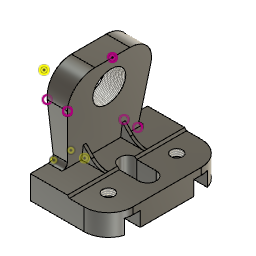
Surprise Checkpoint Q6 v1 (Autodesk Fusion 360 design; units mm, degrees)
Autodesk Fusion 360 part; units mm, degrees
note: some values were not read from the file. Chosen so that the rebuilt part matches the saved one: which face or edge a step refers to; the sign of a taper; which pieces of a blend or face edit are solid.
sketch "Sketch1" plane through (0, 0, 0) normal (0, 1, 0) x (1, 0, 0)
  line L0 (0, 0) -> (0, -24)
  line L1 (0, 0) -> (80, 0)
  line L2 (80, 0) -> (80, -22)
  line L3 (80, -22) -> (40, -22)
  line L4 (0, -24) -> (38, -24)
  line L5 (38, -24) -> (40, -22)
  dimension "d1" = 24
  dimension "d2" = 80
  dimension "d3" = 22
  dimension "d4" = 40
  dimension "d5" = 38
  constraint coincident L0.start L1.start
  constraint vertical L0
  constraint perpendicular L0 L1
  constraint perpendicular L1 L2
  constraint perpendicular L2 L3
  constraint perpendicular L0 L4
  measures "d1" distance of L0.start L0.end
  measures "d2" distance of L0.start L1.end
  measures "d3" distance of L1.end L2.end L0.start
  measures "d4" distance of L2.end L3.end L0.start
  measures "d5" distance of L0.end L4.end
extrude "Extrude1" add sketch "Sketch1" along normal blind 120 makes body 1
fillet "Fillet1" radius 25 2 edges at (80, 0, 11) (80, 120, 11) on bodies 1
hole "Hole1" at (55, 25, 22) direction (0, 0, -1) diameter 12.023 depth 7 tip angle 180 bodies 1
thread "Thread1" "ISO Metric profile 14.0 M14x2 6H"
hole "Hole2" at (55, 95, 22) direction (0, 0, -1) diameter 12.023 depth 7 tip angle 180 bodies 1
thread "Thread2" "ISO Metric profile 14.0 M14x2 6H"
ref_plane "WorkPlane1" through (27.5, 60, 12) normal (0, -1, 0) x (-1, 0, 0)
sketch "Sketch2" plane through (27.5, 60, 12) normal (0, -1, 0) x (1, 0, 0)
  line L0 (27.5, 10) -> (27.5, -12)
  line L1 (27.5, -12) -> (-27.5, -12)
  line L2 (-27.5, -12) -> (-27.5, 12)
  line L3 (-27.5, 12) -> (10.5, 12)
  line L4 (10.5, 12) -> (12.5, 10)
  line L5 (12.5, 10) -> (27.5, 10)
  line L6 (-27.5, -12) -> (-27.5, 97)
  line L7 (-27.5, 97) -> (-3.5, 97)
  line L8 (-27.5, 12) -> (35, 12) construction
  line L9 (-3.5, 97) -> (76.6186, 97) construction
  line L10 (-3.5, 97) -> (82.0862, 97) construction
  line L11 (-3.5, 97) -> (-13.4998, 12)
  line L12 (-3.5, 97) -> (-89.0862, 97) construction
  dimension "d21" = 109
  dimension "d25" = 83.29
  constraint coincident L1.end L2.start
  constraint perpendicular L3 L6
  constraint perpendicular L6 L7
  constraint coincident L2.end L3.start
  constraint perpendicular L2 L8
  constraint horizontal L9
  constraint horizontal L10
  constraint horizontal L12
  constraint coincident L3 L11.end
  measures "d21" distance of L1.end L6.end
  measures "d25" angle of L11 L12
ref_plane "WorkPlane2" through (0, 60, 12) normal (-1, 0, 0) x (0, 0, 1)
sketch "Sketch3" plane through (0, 60, 12) normal (-1, 0, 0) x (0, 1, 0)
ref_plane "WorkPlane3" through (19, 60, 24) normal (0, 0, 1) x (1, 0, 0)
sketch "Sketch4" plane through (0, 0, 24) normal (0, 0, 1) x (-1, 0, 0)
  line L0 (0, 0) -> (-38, 0)
  line L1 (-38, 0) -> (-38, -120)
  line L2 (-38, -120) -> (0, -120)
  line L3 (0, -120) -> (0, 0)
  line L4 (-14.0002, -60) -> (-14.0002, 0)
  line L5 (0, 0) -> (0, -60)
  line L6 (0, -60) -> (0, -30)
  line L7 (0, -60) -> (0, -30)
  point P0 (-14.0002, -60)
  point P1 (0, -60)
  point P2 (0, 0)
  constraint coincident P0 L4.start
  constraint coincident L0 L4.end
  constraint perpendicular L0 L4
  constraint coincident P2 L0.start
  constraint coincident P1 L5.end
  constraint midpoint L5 L6.end
  constraint parallel L6 L7
sketch "Sketch5" plane through (0, 60, 12) normal (-1, 0, 0) x (0, 1, 0)
ref_plane "WorkPlane4" through (24, 60, 109) normal (0, 0, 1) x (1, 0, 0)
sketch "Sketch6" plane through (24, 60, 109) normal (0, 0, 1) x (1, 0, 0)
  point P0 (-24, -45.9998)
ref_plane "WorkPlane5" through (0, 14.0002, 109) normal (0, 0.993151, 0.116837) x (-1, 0, 0)
sketch "Sketch7" plane through (0, 14.0002, 109) normal (0, 0.993151, 0.116837) x (-1, 0, 0)
  point P0 (0, -85.5862)
sweep "Sweep1" add profiles "Sketch2" path "Sketch4" along L5 for 0.59993 of its length starting at (0, 0, 24) heading (0, 1, 0) section 1 contours L3 L6 L7 L11 bodies 1
draft "Draft1" angle 6.71 neutral plane through (0, 14.0002, 109) pull (0, -0.993151, -0.116837) 1 faces at (12.6667, 24.0042, 80.6667) on bodies 1
fillet "Fillet2" radius 25 1 edges at (12, 14, 109) on bodies 1
ref_plane "WorkPlane6" through (24, 60, 109) normal (0, -1, 0) x (1, 0, 0)
sketch "Sketch8" plane through (11.0241, 0, -1.2969) normal (0.993151, 0, -0.116839) x (0, 1, 0)
  ellipse E0 centre (42.1135, 85.8852) end of major axis (42.1135, 111.0576) minor radius 25 (42.1135, 111.0576) -> (17.2848, 82.944) ccw
  line L0 (60, 111.0576) -> (42.1135, 111.0576)
mirror "Mirror1" about plane through (24, 60, 109) normal (0, -1, 0) of bodies 1 makes body 2
combine "Combine1" operation add target body 1 tool bodies 2
sketch "Sketch9" plane through (0, 0, 24) normal (0, 0, 1) x (-1, 0, 0)
  line L0 (0, -96.0002) -> (-14.0002, -96.0002)
sketch "Sketch10" plane through (11.0241, 0, -1.2969) normal (0.993151, 0, -0.116839) x (0, 1, 0)
  ellipse E0 centre (42.1135, 85.8852) end of major axis (42.1135, 111.0576) minor radius 25 (42.1135, 111.0576) -> (17.2848, 82.944) ccw
  line L0 (96.0002, 25.4714) -> (102.7152, 82.944)
  ellipse E1 centre (77.8865, 85.8852) end of major axis (77.8865, 111.0576) minor radius 25 (102.7152, 82.944) -> (77.8865, 111.0576) ccw
  line L1 (77.8865, 111.0576) -> (42.1135, 111.0576)
  point P0 (41.5, 25.4714)
sketch "Sketch11" plane through (0, 0, 24) normal (0, 0, 1) x (-1, 0, 0)
sketch "Sketch12" plane through (0, 0, 22) normal (0, 0, 1) x (-1, 0, 0)
  circle A0 centre (-55, -95) radius 6.0113
  circle A1 centre (-55, -25) radius 6.0113
  arc A2 (-80, -95) -> (-55, -120) centre (-55, -95) ccw
  line L0 (-55, -120) -> (-40, -120)
  line L1 (-40, 0) -> (-55, 0)
  arc A3 (-55, 0) -> (-80, -25) centre (-55, -25) ccw
  line L2 (-80, -25) -> (-80, -95)
  arc A4 (-60, -51) -> (-60, -69) centre (-60, -60) ccw
  line L3 (-60, -51) -> (-57.6575, -51)
  line L4 (-57.6575, -51) -> (-40, -51)
  line L5 (-60, -69) -> (-40, -69)
  arc A5 (-40, -69) -> (-40, -51) centre (-40, -60) ccw
  dimension "d48" = 9
  constraint tangent A4 L5
  measures "d48" radius of A4
extrude "Extrude2" cut sketch "Sketch12" along normal blind 2 and the other way blind 22 contours A4 L3 L4 L5 A5 bodies 1
sketch "Sketch13" plane through (0, 0, 0) normal (-1, 0, 0) x (0, -1, 0)
  arc A0 (-17.2848, 81.079) -> (-42.1135, 109) centre (-42.1135, 84) ccw
  line L0 (-42.1135, 109) -> (-77.8865, 109)
  arc A1 (-77.8865, 109) -> (-102.7152, 81.079) centre (-77.8865, 84) ccw
  line L1 (-102.7152, 81.079) -> (-96.0002, 24)
hole "Hole3" at (0, 60.0039, 81.6923) direction (1, 0, 0) diameter 33.526 depth 30 tip angle 180 bodies 1
thread "Thread3" "ISO Metric profile 35.0 M35x1.5 6H"
fillet "Fillet3" radius 5 1 edges at (7.0001, 96.0002, 24) on bodies 1
fillet "Fillet3" radius 5 1 edges at (7.0001, 23.9998, 24) on bodies 1
sketch "Sketch14" plane through (0, 26.4571, 3.1126) normal (0, -0.993151, -0.116839) x (1, 0, 0)
ref_plane "WorkPlane7" through (14.0002, 41.5, 24) normal (0.993151, 0, -0.116839) x (0, 1, 0)
sketch "Sketch15" plane through (14.0002, 41.5, 24) normal (0.993151, 0, -0.116839) x (0, 1, 0)
ref_plane "WorkPlane8" through (0, 24, 24) normal (-1, 0, 0) x (0, -1, 0)
sketch "Sketch16" plane through (0, 24, 24) normal (-1, 0, 0) x (0, 1, 0)
  point P0 (17.5, 0)
sketch "Sketch17" plane through (14.0002, 41.5, 24) normal (0.993151, 0, -0.116839) x (0, 1, 0)
ref_plane "WorkPlane9" through (0, 41.5, 24) normal (0, 1, 0) x (-1, 0, 0)
sketch "Sketch18" plane through (0, 41.5, 24) normal (0, 1, 0) x (1, 0, 0)
  point P0 (14.0002, 0)
sketch "Sketch19" plane through (0, 0, 24) normal (0, 0, 1) x (1, 0, 0)
sketch "Sketch20" plane through (0, 0, 24) normal (0, 0, 1) x (1, 0, 0)
sketch "Sketch21" plane through (0, 41.5, 24) normal (0, 1, 0) x (1, 0, 0)
  line L0 (14.0002, 0) -> (38, 0)
  line L1 (26.4, 0) -> (26.4, 24)
  line L2 (38, 0) -> (38, 23.5536)
  line L3 (41.2843, -45) -> (43.8884, -45) construction
  line L4 (4.7157, -25) -> (6.6099, -23.1058)
  line L5 (4.7157, -25) -> (-13.0247, -25) construction
  line L6 (24, -85) -> (14.0002, 0)
  line L7 (15.6429, -13.9635) -> (14.0002, 0)
  line L8 (26.4, 0) -> (14.0002, 0)
  line L9 (29.7157, 0) -> (26.4, 0)
  line L10 (29.7157, 0) -> (26.4, 0)
  line L11 (15.6429, -13.9635) -> (14.0002, 0)
  line L12 (14.0002, 0) -> (29.7157, 0)
  line L13 (15.6544, -14.0613) -> (4.7157, -25)
  arc A0 (38, 0) -> (23.8579, -5.8579) centre (38, -20) ccw
  line L14 (15.6544, -14.0613) -> (23.8579, -5.8579)
  point P0 (14.0002, 0)
  dimension "d63" = 40
  dimension "d65" = 45
  constraint coincident L1.start L8.start
  constraint perpendicular L0 L1
  constraint tangent L0 A0
  constraint coincident L0.end L2.start
  constraint perpendicular L0 L2
  constraint collinear A0.centre L0.end L2.end
  constraint horizontal L3
  constraint horizontal L5
  constraint tangent L4 A0
  constraint coincident L6 L7.start
  constraint coincident P0 L0.start
  constraint parallel L6 L7
  constraint coincident L0 L9.start
  constraint perpendicular L1 L9
  constraint parallel L0 L12
  constraint coincident L6 L13.start
  constraint tangent A0 L14
  measures "d63" diameter of A0
  measures "d65" angle of L4 L5
extrude "Extrude3" add sketch "Sketch21" against normal blind 3 bodies 1
mirror "Mirror2" about plane through (24, 60, 109) normal (0, -1, 0) of bodies 1 makes body 3
sketch "Sketch22" plane through (80, 0, 0) normal (1, 0, 0) x (0, 1, 0)
  line L0 (25, 22) -> (25, 0)
  line L1 (25, 0) -> (95, 0)
  line L2 (95, 0) -> (95, 22)
  line L3 (95, 22) -> (25, 22)
  line L4 (0, 0) -> (17.5, 0)
  line L5 (0, 0) -> (32.5, 0)
  line L6 (17.5, 0) -> (17.5, 15)
  line L7 (32.5, 0) -> (32.5, 15)
  line L8 (32.5, 15) -> (17.5, 15)
  dimension "d69" = 17.5
  dimension "d70" = 32.5
  dimension "d71" = 15
  constraint coincident L4.start L5.start
  constraint horizontal L4
  constraint coincident L1 L5.end
  constraint perpendicular L4 L6
  constraint perpendicular L5 L7
  constraint perpendicular L6 L8
  measures "d69" distance of L4.start L4.end
  measures "d70" distance of L4.start L5.end
  measures "d71" distance of L4.end L6.end
extrude "Extrude4" cut sketch "Sketch22" against normal blind 25 contours L0 L1 L5 L7 L8 | L0 L5 L6 L8 bodies 1 3
sketch "Sketch23" plane through (80, 0, 0) normal (1, 0, 0) x (0, 1, 0)
  line L0 (32.5, 15) -> (32.5, 0)
  line L1 (32.5, 0) -> (95, 0)
  line L2 (95, 0) -> (95, 22)
  line L3 (95, 22) -> (25, 22)
  line L4 (25, 22) -> (25, 15)
  line L5 (25, 15) -> (32.5, 15)
  line L6 (0, 0) -> (87.5, 0)
  line L7 (0, 0) -> (102.5, 0)
  line L8 (87.5, 0) -> (87.5, 15)
  line L9 (87.5, 15) -> (102.5, 15)
  line L10 (102.5, 15) -> (102.5, 0)
  dimension "d74" = 87.5
  dimension "d75" = 102.5
  constraint coincident L6.start L7.start
  constraint perpendicular L0 L6
  constraint parallel L6 L7
  constraint perpendicular L7 L8
  constraint perpendicular L2 L9
  constraint perpendicular L7 L10
  measures "d74" distance of L6.start L6.end
  measures "d75" distance of L6.start L7.end
extrude "Extrude5" cut sketch "Sketch23" against normal blind 25 contours L1 L2 L7 L8 L9 | L2 L7 L9 L10 bodies 1 3
